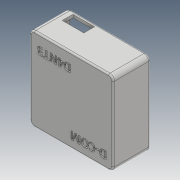
# Autodesk Inventor part: base
Saved by Autodesk Inventor 2017 (Build 210142000, 142)
## iProperties
Created: 2020-06-11
Part Number: base
Material: Generic
Document SubType Name: Modeling
Designer: c
Density: 1 g/cm^3
Appearance: Default
Author: c
Autodesk Inventor part; units mm, degrees
ref_plane "YZ Plane" through (0, 0, 0) normal (1, 0, 0) x (0, 1, 0)
ref_plane "XZ Plane" through (0, 0, 0) normal (0, 1, 0) x (-1, 0, 0)
ref_plane "XY Plane" through (0, 0, 0) normal (0, 0, 1) x (1, 0, 0)
sketch "Sketch1" plane through (0, 0, 0) normal (0, 1, 0) x (-1, 0, 0)
  line L0 (13, 15) -> (-37, 15)
  line L1 (-37, 15) -> (-37, -35)
  line L2 (-37, -35) -> (13, -35)
  line L3 (13, -35) -> (13, 15)
  line L4 (12, 17) -> (-36, 17)
  line L5 (-39, 14) -> (-39, -34)
  line L6 (-36, -37) -> (12, -37)
  line L7 (15, -34) -> (15, 14)
  arc A0 (15, 14) -> (12, 17) centre (12, 14) ccw
  arc A1 (-36, 17) -> (-39, 14) centre (-36, 14) ccw
  arc A2 (-39, -34) -> (-36, -37) centre (-36, -34) ccw
  arc A3 (12, -37) -> (15, -34) centre (12, -34) ccw
  point P0 (0, 0)
  dimension "d0" = 50
  dimension "d1" = 50
  dimension "d2" = 3
  constraints: 16 end point, 8 point on circle, 8 tangent, 4 centre point, 4 parallel, 3 equal radius, 2 perpendicular, 1 horizontal, 3 other
  measures "d0" distance of L2.end L1.end
  measures "d1" distance of L1.end L0.end
  measures "d2" radius of A0
extrude "Extrusion1" add sketch "Sketch1" along normal blind 24
sketch "Sketch2" plane through (0, 0, 0) normal (0, -1, 0) x (1, 0, 0)
  line L0 (36, 17) -> (-12, 17)
  line L1 (-15, 14) -> (-15, -34)
  line L2 (-12, -37) -> (36, -37)
  line L3 (39, -34) -> (39, 14)
  arc A0 (39, 14) -> (36, 17) centre (36, 14) ccw
  arc A1 (-12, 17) -> (-15, 14) centre (-12, 14) ccw
  arc A2 (-15, -34) -> (-12, -37) centre (-12, -34) ccw
  arc A3 (36, -37) -> (39, -34) centre (36, -34) ccw
  point P0 (0, 0)
  dimension "d5" = 3
  constraints: 8 end point, 8 point on circle, 8 tangent, 4 centre point, 3 equal radius, 2 parallel, 1 horizontal, 1 perpendicular
  measures "d5" radius of A0
extrude "Extrusion2" add sketch "Sketch2" against normal blind 2
fillet "Fillet1" radius 1 8 edges at (-14.1213, 0, 16.1213) (-15, 0, -10) (-14.1213, 0, -36.1213) (12, 0, -37) (38.1213, 0, -36.1213) (39, 0, -10) (38.1213, 0, 16.1213) (12, 0, 17)
sketch "Sketch3" plane through (36, 24, -37) normal (0, 0, -1) x (-1, 0, 0)
  line L0 (29, -12) -> (19, -12)
  line L1 (19, -12) -> (19, -8)
  line L2 (19, -8) -> (29, -8)
  line L3 (29, -8) -> (29, -12)
  line L4 (29, -18) -> (19, -18)
  line L5 (19, -18) -> (19, -14)
  line L6 (19, -14) -> (29, -14)
  line L7 (29, -14) -> (29, -18)
  line L8 (0, 0) -> (48, 0) projected
  line L9 (51, -23) -> (51, 0) projected
  line L10 (0, -24) -> (48, -24) projected
  point P0 (36, -24)
  dimension "d9" = 10
  dimension "d10" = 4
  dimension "d11" = 10
  dimension "d12" = 2
  dimension "d16" = 22
  dimension "d17" = 4
  dimension "d25" = 10
  constraints: 16 end point, 4 parallel, 2 horizontal, 2 perpendicular, 1 point on line
  measures "d9" distance of L1.end L2.end
  measures "d10" distance of L0.end L1.end
  measures "d11" distance of L5.end L6.end
  measures "d12" distance between parallel lines of L0 L6
  measures "d16" distance between parallel lines of L9 L7
  measures "d17" distance of L4.end L5.end
  measures "d25" distance between parallel lines of L10 L6
extrude "Extrusion3" cut sketch "Sketch3" against normal blind 4
sketch "Sketch4" plane through (0, 0, 0) normal (0, -1, 0) x (1, 0, 0)
  line L0 (11.8173, 5.1202) -> (-9.0886, 5.1202) construction
  line L1 (-9.0886, 5.1202) -> (-9.0886, 15.4837) construction
  line L2 (-9.0886, 15.4837) -> (11.8173, 15.4837) construction
  line L3 (11.8173, 15.4837) -> (11.8173, 5.1202) construction
  line L4 (34.9838, -32.0104) -> (14.0779, -32.0104) construction
  line L5 (14.0779, -32.0104) -> (14.0779, 11.03) construction
  line L6 (14.0779, 11.03) -> (34.9838, 11.03) construction
  line L7 (34.9838, 11.03) -> (34.9838, -32.0104) construction
  spline S0 degree 2 poles (7.1365, 7.6225) (7.1365, 8.3079) (7.4933, 9.2798) (8.1647, 9.8995) (9.1224, 10.1859) (9.7844, 10.1859) knots 0 0 0 1 2 3 4 4 4
  line L8 (9.7844, 10.1859) -> (10.9722, 10.1859)
  spline S1 degree 2 poles (10.9722, 10.1859) (11.0989, 10.1859) (11.2727, 10.0356) (11.2727, 9.8666) knots 0 0 0 1 2 2 2
  line L9 (11.2727, 9.8666) -> (11.2727, 5.5286)
  spline S2 degree 2 poles (11.2727, 5.5286) (11.2727, 5.3596) (11.0989, 5.2094) (10.9722, 5.2094) knots 0 0 0 1 2 2 2
  line L10 (10.9722, 5.2094) -> (9.6952, 5.2094)
  spline S3 degree 2 poles (9.6952, 5.2094) (9.0285, 5.2094) (8.1036, 5.5192) (7.4651, 6.1342) (7.1365, 7.031) (7.1365, 7.6225) knots 0 0 0 1 2 3 4 4 4
  spline S4 degree 2 poles (8.1835, 7.6601) (8.1835, 7.3079) (8.3478, 6.6976) (8.714, 6.2516) (9.2867, 6.0028) (9.7515, 6.0028) knots 0 0 0 1 2 3 4 4 4
  line L11 (9.7515, 6.0028) -> (10.2633, 6.0028)
  line L12 (10.2633, 6.0028) -> (10.2633, 9.3878)
  line L13 (10.2633, 9.3878) -> (9.7374, 9.3878)
  spline S5 degree 2 poles (9.7374, 9.3878) (9.3196, 9.3878) (8.7515, 9.1718) (8.3712, 8.7399) (8.1835, 8.092) (8.1835, 7.6601) knots 0 0 0 1 2 3 4 4 4
  spline S6 degree 2 poles (3.0144, 8.7587) (3.0144, 8.9558) (3.0942, 9.1577) (3.1647, 9.1577) knots 0 0 0 1 2 2 2
  line L14 (3.1647, 9.1577) -> (3.606, 9.1577)
  line L15 (3.606, 9.1577) -> (3.606, 10.0544)
  spline S7 degree 2 poles (3.606, 10.0544) (3.606, 10.092) (3.6529, 10.153) (3.7656, 10.1906) (3.9534, 10.2094) (4.0989, 10.2094) knots 0 0 0 1 2 3 4 4 4
  spline S8 degree 2 poles (4.0989, 10.2094) (4.2351, 10.2094) (4.4229, 10.1906) (4.5356, 10.153) (4.5778, 10.092) (4.5778, 10.0544) knots 0 0 0 1 2 3 4 4 4
  line L16 (4.5778, 10.0544) -> (4.5778, 9.1577)
  line L17 (4.5778, 9.1577) -> (6.4839, 9.1577)
  spline S9 degree 2 poles (6.4839, 9.1577) (6.5403, 9.1577) (6.6248, 9.1295) (6.6811, 9.0356) (6.7093, 8.8525) (6.7093, 8.7023) knots 0 0 0 1 2 3 4 4 4
  spline S10 degree 2 poles (6.7093, 8.7023) (6.7093, 8.5802) (6.6999, 8.4018) (6.6717, 8.2516) (6.6201, 8.1248) (6.5825, 8.0497) knots 0 0 0 1 2 3 4 4 4
  line L18 (6.5825, 8.0497) -> (5.0332, 5.322)
  spline S11 degree 2 poles (5.0332, 5.322) (5.0144, 5.2845) (4.9205, 5.2375) (4.7562, 5.2) (4.5027, 5.1859) (4.3196, 5.1859) knots 0 0 0 1 2 3 4 4 4
  spline S12 degree 2 poles (4.3196, 5.1859) (4.1224, 5.1859) (3.8501, 5.2047) (3.6811, 5.2469) (3.606, 5.3079) (3.606, 5.3502) knots 0 0 0 1 2 3 4 4 4
  line L19 (3.606, 5.3502) -> (3.606, 8.3502)
  line L20 (3.606, 8.3502) -> (3.1647, 8.3502)
  spline S13 degree 2 poles (3.1647, 8.3502) (3.1036, 8.3502) (3.0144, 8.538) (3.0144, 8.7587) knots 0 0 0 1 2 2 2
  line L21 (4.5778, 6.0591) -> (4.5872, 6.0591)
  line L22 (4.5872, 6.0591) -> (5.9018, 8.3502)
  line L23 (5.9018, 8.3502) -> (4.5778, 8.3502)
  line L24 (4.5778, 8.3502) -> (4.5778, 6.0591)
  spline S14 degree 2 poles (-1.7884, 9.8338) (-1.7884, 9.923) (-1.7273, 10.0591) (-1.6241, 10.153) (-1.4785, 10.1953) (-1.4081, 10.1953) knots 0 0 0 1 2 3 4 4 4
  line L25 (-1.4081, 10.1953) -> (-0.9762, 10.1953)
  spline S15 degree 2 poles (-0.9762, 10.1953) (-0.8447, 10.1953) (-0.6475, 10.1389) (-0.4832, 9.9981) (-0.3283, 9.754) (-0.2297, 9.5662) knots 0 0 0 1 2 3 4 4 4
  line L26 (-0.2297, 9.5662) -> (1.0097, 7.2375)
  spline S16 degree 2 poles (1.0097, 7.2375) (1.1177, 7.031) (1.3384, 6.5474) (1.4276, 6.322) knots 0 0 0 1 2 2 2
  line L27 (1.4276, 6.322) -> (1.437, 6.322)
  spline S17 degree 2 poles (1.437, 6.322) (1.4182, 6.599) (1.4041, 7.1483) (1.4041, 7.4394) knots 0 0 0 1 2 2 2
  line L28 (1.4041, 7.4394) -> (1.4041, 10.045)
  spline S18 degree 2 poles (1.4041, 10.045) (1.4041, 10.0826) (1.4464, 10.1436) (1.5496, 10.1859) (1.7281, 10.2094) (1.8642, 10.2094) knots 0 0 0 1 2 3 4 4 4
  spline S19 degree 2 poles (1.8642, 10.2094) (2.0004, 10.2094) (2.1788, 10.1859) (2.2773, 10.1436) (2.3149, 10.0826) (2.3149, 10.045) knots 0 0 0 1 2 3 4 4 4
  line L29 (2.3149, 10.045) -> (2.3149, 5.5709)
  spline S20 degree 2 poles (2.3149, 5.5709) (2.3149, 5.3878) (2.1036, 5.2094) (1.9487, 5.2094) knots 0 0 0 1 2 2 2
  line L30 (1.9487, 5.2094) -> (1.4088, 5.2094)
  spline S21 degree 2 poles (1.4088, 5.2094) (1.2633, 5.2094) (1.0614, 5.261) (0.9065, 5.3737) (0.7656, 5.5802) (0.6905, 5.7305) knots 0 0 0 1 2 3 4 4 4
  line L31 (0.6905, 5.7305) -> (-0.2766, 7.5474)
  spline S22 degree 2 poles (-0.2766, 7.5474) (-0.3611, 7.7164) (-0.5255, 8.0356) (-0.6804, 8.3549) (-0.8259, 8.6601) (-0.8964, 8.815) knots 0 0 0 1 2 3 4 4 4
  line L32 (-0.8964, 8.815) -> (-0.9011, 8.815)
  spline S23 degree 2 poles (-0.9011, 8.815) (-0.887, 8.5474) (-0.8776, 7.9605) (-0.8776, 7.6929) knots 0 0 0 1 2 2 2
  line L33 (-0.8776, 7.6929) -> (-0.8776, 5.3549)
  spline S24 degree 2 poles (-0.8776, 5.3549) (-0.8776, 5.3173) (-0.9245, 5.2563) (-1.0325, 5.2094) (-1.2062, 5.1906) (-1.3471, 5.1906) knots 0 0 0 1 2 3 4 4 4
  spline S25 degree 2 poles (-1.3471, 5.1906) (-1.4785, 5.1906) (-1.6522, 5.2094) (-1.7508, 5.2563) (-1.7884, 5.3173) (-1.7884, 5.3549) knots 0 0 0 1 2 3 4 4 4
  line L34 (-1.7884, 5.3549) -> (-1.7884, 9.8338)
  spline S26 degree 2 poles (-6.1781, 5.6225) (-6.1781, 5.7352) (-6.1593, 5.8948) (-6.1217, 5.9887) (-6.0607, 6.0356) (-6.0278, 6.0356) knots 0 0 0 1 2 3 4 4 4
  line L35 (-6.0278, 6.0356) -> (-4.7837, 6.0356)
  line L36 (-4.7837, 6.0356) -> (-4.7837, 10.0497)
  spline S27 degree 2 poles (-4.7837, 10.0497) (-4.7837, 10.0873) (-4.732, 10.1483) (-4.6194, 10.1859) (-4.4222, 10.2094) (-4.2766, 10.2094) knots 0 0 0 1 2 3 4 4 4
  spline S28 degree 2 poles (-4.2766, 10.2094) (-4.1311, 10.2094) (-3.9339, 10.1859) (-3.8212, 10.1483) (-3.7696, 10.0873) (-3.7696, 10.0497) knots 0 0 0 1 2 3 4 4 4
  line L37 (-3.7696, 10.0497) -> (-3.7696, 6.0356)
  line L38 (-3.7696, 6.0356) -> (-2.5255, 6.0356)
  spline S29 degree 2 poles (-2.5255, 6.0356) (-2.4879, 6.0356) (-2.4316, 5.9887) (-2.394, 5.8948) (-2.3752, 5.7352) (-2.3752, 5.6225) knots 0 0 0 1 2 3 4 4 4
  spline S30 degree 2 poles (-2.3752, 5.6225) (-2.3752, 5.5098) (-2.394, 5.3455) (-2.4316, 5.2516) (-2.4879, 5.2094) (-2.5255, 5.2094) knots 0 0 0 1 2 3 4 4 4
  line L39 (-2.5255, 5.2094) -> (-6.0278, 5.2094)
  spline S31 degree 2 poles (-6.0278, 5.2094) (-6.0607, 5.2094) (-6.1217, 5.2516) (-6.1593, 5.3455) (-6.1781, 5.5098) (-6.1781, 5.6225) knots 0 0 0 1 2 3 4 4 4
  spline S32 degree 2 poles (-9.887, 8.7305) (-9.887, 9.1014) (-9.6006, 9.6788) (-9.0935, 10.0732) (-8.3846, 10.2751) (-7.9668, 10.2751) knots 0 0 0 1 2 3 4 4 4
  spline S33 degree 2 poles (-7.9668, 10.2751) (-7.7133, 10.2751) (-7.2673, 10.2) (-6.9245, 10.0967) (-6.6992, 9.9793) (-6.6335, 9.9183) (-6.5959, 9.8385) (-6.5677, 9.7352) (-6.5583, 9.5802) (-6.5583, 9.4676) knots 0 0 0 1 2 3 4 5 6 7 8 8 8
  spline S34 degree 2 poles (-6.5583, 9.4676) (-6.5583, 9.2798) (-6.6194, 9.1389) (-6.6804, 9.1389) knots 0 0 0 1 2 2 2
  spline S35 degree 2 poles (-6.6804, 9.1389) (-6.718, 9.1389) (-6.9104, 9.2422) (-7.2015, 9.3643) (-7.5959, 9.4676) (-7.8447, 9.4676) knots 0 0 0 1 2 3 4 4 4
  spline S36 degree 2 poles (-7.8447, 9.4676) (-8.056, 9.4676) (-8.3799, 9.369) (-8.6053, 9.1859) (-8.718, 8.9277) (-8.718, 8.7727) knots 0 0 0 1 2 3 4 4 4
  spline S37 degree 2 poles (-8.718, 8.7727) (-8.718, 8.599) (-8.5818, 8.322) (-8.3189, 8.1248) (-7.9151, 8.0169) (-7.6381, 8.0169) knots 0 0 0 1 2 3 4 4 4
  line L40 (-7.6381, 8.0169) -> (-7.2062, 8.0169)
  spline S38 degree 2 poles (-7.2062, 8.0169) (-7.1593, 8.0169) (-7.0888, 7.9887) (-7.0419, 7.9042) (-7.0231, 7.754) (-7.0231, 7.6366) knots 0 0 0 1 2 3 4 4 4
  spline S39 degree 2 poles (-7.0231, 7.6366) (-7.0231, 7.5239) (-7.0419, 7.3831) (-7.0842, 7.3079) (-7.1499, 7.2751) (-7.1968, 7.2751) knots 0 0 0 1 2 3 4 4 4
  line L41 (-7.1968, 7.2751) -> (-7.6335, 7.2751)
  spline S40 degree 2 poles (-7.6335, 7.2751) (-7.8588, 7.2751) (-8.2062, 7.1718) (-8.441, 6.9793) (-8.563, 6.707) (-8.563, 6.538) knots 0 0 0 1 2 3 4 4 4
  spline S41 degree 2 poles (-8.563, 6.538) (-8.563, 6.4112) (-8.4785, 6.1859) (-8.3142, 6.0216) (-8.0513, 5.923) (-7.8729, 5.923) knots 0 0 0 1 2 3 4 4 4
  spline S42 degree 2 poles (-7.8729, 5.923) (-7.671, 5.923) (-7.3189, 6.0403) (-7.0372, 6.1859) (-6.84, 6.3079) (-6.7931, 6.3079) knots 0 0 0 1 2 3 4 4 4
  spline S43 degree 2 poles (-6.7931, 6.3079) (-6.7649, 6.3079) (-6.718, 6.2798) (-6.6851, 6.2047) (-6.671, 6.0591) (-6.671, 5.9417) knots 0 0 0 1 2 3 4 4 4
  spline S44 degree 2 poles (-6.671, 5.9417) (-6.671, 5.8479) (-6.6804, 5.7211) (-6.7039, 5.6366) (-6.7367, 5.5756) (-6.8119, 5.5004) (-7.0513, 5.3549) (-7.4128, 5.214) (-7.887, 5.1202) (-8.164, 5.1202) knots 0 0 0 1 2 3 4 5 6 7 8 8 8
  spline S45 degree 2 poles (-8.164, 5.1202) (-8.5255, 5.1202) (-9.0842, 5.2892) (-9.4644, 5.6084) (-9.6616, 6.0732) (-9.6616, 6.369) knots 0 0 0 1 2 3 4 4 4
  spline S46 degree 2 poles (-9.6616, 6.369) (-9.6616, 6.5943) (-9.5442, 6.984) (-9.3236, 7.2939) (-8.9856, 7.5098) (-8.7696, 7.5615) knots 0 0 0 1 2 3 4 4 4
  line L42 (-8.7696, 7.5615) -> (-8.7696, 7.5756)
  spline S47 degree 2 poles (-8.7696, 7.5756) (-9.0278, 7.6037) (-9.4457, 7.8103) (-9.732, 8.1155) (-9.887, 8.5051) (-9.887, 8.7305) knots 0 0 0 1 2 3 4 4 4
  spline S48 degree 2 poles (30.303, -29.5081) (30.303, -28.8226) (30.6598, -27.8508) (31.3312, -27.2311) (32.2889, -26.9447) (32.9509, -26.9447) knots 0 0 0 1 2 3 4 4 4
  line L43 (32.9509, -26.9447) -> (34.1387, -26.9447)
  spline S49 degree 2 poles (34.1387, -26.9447) (34.2654, -26.9447) (34.4392, -27.0949) (34.4392, -27.2639) knots 0 0 0 1 2 2 2
  line L44 (34.4392, -27.2639) -> (34.4392, -31.602)
  spline S50 degree 2 poles (34.4392, -31.602) (34.4392, -31.771) (34.2654, -31.9212) (34.1387, -31.9212) knots 0 0 0 1 2 2 2
  line L45 (34.1387, -31.9212) -> (32.8617, -31.9212)
  spline S51 degree 2 poles (32.8617, -31.9212) (32.195, -31.9212) (31.2701, -31.6114) (30.6316, -30.9963) (30.303, -30.0996) (30.303, -29.5081) knots 0 0 0 1 2 3 4 4 4
  spline S52 degree 2 poles (31.35, -29.4705) (31.35, -29.8226) (31.5143, -30.433) (31.8805, -30.879) (32.4532, -31.1278) (32.918, -31.1278) knots 0 0 0 1 2 3 4 4 4
  line L46 (32.918, -31.1278) -> (33.4298, -31.1278)
  line L47 (33.4298, -31.1278) -> (33.4298, -27.7428)
  line L48 (33.4298, -27.7428) -> (32.9039, -27.7428)
  spline S53 degree 2 poles (32.9039, -27.7428) (32.4861, -27.7428) (31.918, -27.9588) (31.5377, -28.3907) (31.35, -29.0386) (31.35, -29.4705) knots 0 0 0 1 2 3 4 4 4
  spline S54 degree 2 poles (27.8335, -28.879) (27.8335, -28.6583) (27.918, -28.4799) (28.0119, -28.4799) knots 0 0 0 1 2 2 2
  line L49 (28.0119, -28.4799) -> (29.6082, -28.4799)
  spline S55 degree 2 poles (29.6082, -28.4799) (29.7068, -28.4799) (29.7913, -28.663) (29.7913, -28.879) knots 0 0 0 1 2 2 2
  spline S56 degree 2 poles (29.7913, -28.879) (29.7913, -29.0949) (29.7068, -29.2733) (29.6082, -29.2733) knots 0 0 0 1 2 2 2
  line L50 (29.6082, -29.2733) -> (28.0119, -29.2733)
  spline S57 degree 2 poles (28.0119, -29.2733) (27.965, -29.2733) (27.8992, -29.2358) (27.8523, -29.1419) (27.8335, -28.9869) (27.8335, -28.879) knots 0 0 0 1 2 3 4 4 4
  spline S58 degree 2 poles (23.6176, -27.7006) (23.6176, -27.6067) (23.6269, -27.4705) (23.6504, -27.3766) (23.6927, -27.3062) (23.7772, -27.217) (24.0166, -27.0761) (24.3687, -26.9494) (24.8194, -26.8649) (25.0777, -26.8649) knots 0 0 0 1 2 3 4 5 6 7 8 8 8
  spline S59 degree 2 poles (25.0777, -26.8649) (25.5894, -26.8649) (26.4157, -27.1794) (26.9885, -27.8085) (27.2983, -28.7428) (27.2983, -29.3672) knots 0 0 0 1 2 3 4 4 4
  spline S60 degree 2 poles (27.2983, -29.3672) (27.2983, -30.001) (26.9603, -30.9869) (26.35, -31.6536) (25.5002, -32.001) (24.9885, -32.001) knots 0 0 0 1 2 3 4 4 4
  spline S61 degree 2 poles (24.9885, -32.001) (24.7819, -32.001) (24.3969, -31.9306) (24.0683, -31.8179) (23.81, -31.6724) (23.7068, -31.5691) (23.6645, -31.4987) (23.641, -31.3907) (23.6316, -31.2452) (23.6316, -31.1372) knots 0 0 0 1 2 3 4 5 6 7 8 8 8
  spline S62 degree 2 poles (23.6316, -31.1372) (23.6316, -31.0245) (23.6457, -30.8602) (23.6833, -30.7616) (23.7396, -30.7146) (23.7725, -30.7146) knots 0 0 0 1 2 3 4 4 4
  spline S63 degree 2 poles (23.7725, -30.7146) (23.8335, -30.7146) (24.0072, -30.8508) (24.2889, -31.0151) (24.6786, -31.1513) (24.9462, -31.1513) knots 0 0 0 1 2 3 4 4 4
  spline S64 degree 2 poles (24.9462, -31.1513) (25.242, -31.1513) (25.7068, -30.9071) (26.0354, -30.4611) (26.2044, -29.8226) (26.2044, -29.4236) knots 0 0 0 1 2 3 4 4 4
  spline S65 degree 2 poles (26.2044, -29.4236) (26.2044, -28.9822) (26.026, -28.3437) (25.688, -27.9259) (25.2185, -27.724) (24.9227, -27.724) knots 0 0 0 1 2 3 4 4 4
  spline S66 degree 2 poles (24.9227, -27.724) (24.6504, -27.724) (24.2608, -27.8508) (23.9791, -28.0057) (23.796, -28.1278) (23.749, -28.1278) knots 0 0 0 1 2 3 4 4 4
  spline S67 degree 2 poles (23.749, -28.1278) (23.7115, -28.1278) (23.6645, -28.0949) (23.6316, -28.0057) (23.6176, -27.8414) (23.6176, -27.7006) knots 0 0 0 1 2 3 4 4 4
  spline S68 degree 2 poles (18.411, -29.4893) (18.411, -28.8696) (18.7208, -27.893) (19.3265, -27.2123) (20.2232, -26.8555) (20.81, -26.8555) knots 0 0 0 1 2 3 4 4 4
  spline S69 degree 2 poles (20.81, -26.8555) (21.3922, -26.8555) (22.2608, -27.1607) (22.8382, -27.7804) (23.1246, -28.7428) (23.1246, -29.4001) knots 0 0 0 1 2 3 4 4 4
  spline S70 degree 2 poles (23.1246, -29.4001) (23.1246, -30.0057) (22.8147, -30.9729) (22.2091, -31.6489) (21.3124, -32.0104) (20.7208, -32.0104) knots 0 0 0 1 2 3 4 4 4
  spline S71 degree 2 poles (20.7208, -32.0104) (20.1528, -32.0104) (19.2889, -31.7099) (18.7068, -31.0855) (18.411, -30.1372) (18.411, -29.4893) knots 0 0 0 1 2 3 4 4 4
  spline S72 degree 2 poles (19.472, -29.4376) (19.472, -29.8273) (19.5941, -30.4705) (19.8899, -30.9306) (20.3828, -31.1794) (20.7537, -31.1794) knots 0 0 0 1 2 3 4 4 4
  spline S73 degree 2 poles (20.7537, -31.1794) (21.1293, -31.1794) (21.6269, -30.8977) (21.9368, -30.4283) (22.0636, -29.8038) (22.0636, -29.4517) knots 0 0 0 1 2 3 4 4 4
  spline S74 degree 2 poles (22.0636, -29.4517) (22.0636, -29.0433) (21.9415, -28.3954) (21.6457, -27.9353) (21.1528, -27.6912) (20.7819, -27.6912) knots 0 0 0 1 2 3 4 4 4
  spline S75 degree 2 poles (20.7819, -27.6912) (20.4063, -27.6912) (19.9086, -27.9682) (19.5988, -28.447) (19.472, -29.0808) (19.472, -29.4376) knots 0 0 0 1 2 3 4 4 4
  spline S76 degree 2 poles (11.7584, -27.0808) (11.7584, -27.0433) (11.8007, -26.9822) (11.9133, -26.9447) (12.0964, -26.9212) (12.2373, -26.9212) knots 0 0 0 1 2 3 4 4 4
  spline S77 degree 2 poles (12.2373, -26.9212) (12.3781, -26.9212) (12.5612, -26.9447) (12.6692, -26.9822) (12.7162, -27.0433) (12.7162, -27.0808) knots 0 0 0 1 2 3 4 4 4
  line L51 (12.7162, -27.0808) -> (12.7162, -31.1325)
  line L52 (12.7162, -31.1325) -> (12.7255, -31.1325)
  line L53 (12.7255, -31.1325) -> (14.1669, -27.0855)
  spline S78 degree 2 poles (14.1669, -27.0855) (14.1809, -27.0386) (14.2514, -26.9729) (14.3687, -26.9306) (14.5565, -26.9212) (14.688, -26.9212) knots 0 0 0 1 2 3 4 4 4
  spline S79 degree 2 poles (14.688, -26.9212) (14.8147, -26.9212) (15.0025, -26.94) (15.1199, -26.9822) (15.1903, -27.0433) (15.1997, -27.0855) knots 0 0 0 1 2 3 4 4 4
  line L54 (15.1997, -27.0855) -> (16.5941, -31.1325)
  line L55 (16.5941, -31.1325) -> (16.6035, -31.1325)
  line L56 (16.6035, -31.1325) -> (16.6035, -27.0808)
  spline S80 degree 2 poles (16.6035, -27.0808) (16.6035, -27.0433) (16.6457, -26.9822) (16.7631, -26.9447) (16.9415, -26.9212) (17.0823, -26.9212) knots 0 0 0 1 2 3 4 4 4
  spline S81 degree 2 poles (17.0823, -26.9212) (17.2232, -26.9212) (17.4063, -26.9447) (17.519, -26.9822) (17.5612, -27.0433) (17.5612, -27.0808) knots 0 0 0 1 2 3 4 4 4
  line L57 (17.5612, -27.0808) -> (17.5612, -31.5175)
  spline S82 degree 2 poles (17.5612, -31.5175) (17.5612, -31.7146) (17.3546, -31.9212) (17.1809, -31.9212) knots 0 0 0 1 2 2 2
  line L58 (17.1809, -31.9212) -> (16.519, -31.9212)
  spline S83 degree 2 poles (16.519, -31.9212) (16.3406, -31.9212) (16.087, -31.8649) (15.9039, -31.7287) (15.7819, -31.5081) (15.7349, -31.3484) knots 0 0 0 1 2 3 4 4 4
  line L59 (15.7349, -31.3484) -> (14.6551, -28.3813)
  line L60 (14.6551, -28.3813) -> (14.641, -28.3813)
  line L61 (14.641, -28.3813) -> (13.5237, -31.3391)
  spline S84 degree 2 poles (13.5237, -31.3391) (13.472, -31.5034) (13.3546, -31.724) (13.195, -31.8649) (12.9838, -31.9212) (12.8382, -31.9212) knots 0 0 0 1 2 3 4 4 4
  line L62 (12.8382, -31.9212) -> (12.1575, -31.9212)
  spline S85 degree 2 poles (12.1575, -31.9212) (12.0542, -31.9212) (11.9039, -31.8696) (11.81, -31.7616) (11.7584, -31.6114) (11.7584, -31.5175) knots 0 0 0 1 2 3 4 4 4
  line L63 (11.7584, -31.5175) -> (11.7584, -27.0808)
  point P0 (0, 0)
  constraints: 4 other
emboss "Emboss1" sketch "Sketch4" operation cut depth 1 direction (0, 1, 0)
sketch "Sketch5" plane through (-12, 24, 17) normal (0, 0, 1) x (1, 0, 0)
  line L0 (29, -12) -> (29, -8) projected
  line L1 (17, -9) -> (2.9977, -9)
  line L2 (2.9977, -9) -> (2.9977, -2)
  line L3 (2.9977, -2) -> (17, -2)
  line L4 (17, -2) -> (17, -9)
  line L5 (-3, -23) -> (-3, 0) projected
  line L6 (0, -24) -> (48, -24) projected
  point P0 (12, -24)
  dimension "d26" = 20
  dimension "d27" = 15
  dimension "d28" = 7
  constraints: 8 end point, 2 parallel, 1 horizontal, 1 perpendicular
  measures "d26" distance between parallel lines of L5 L4
  measures "d27" distance between parallel lines of L6 L1
  measures "d28" distance between parallel lines of L1 L3
extrude "Extrusion4" cut sketch "Sketch5" against normal blind 4
fillet "Fillet2" radius 1 8 edges at (38.1213, 24, 16.1213) (39, 24, -10) (38.1213, 24, -36.1213) (12, 24, -37) (-14.1213, 24, -36.1213) (-15, 24, -10) (-14.1213, 24, 16.1213) (12, 24, 17)
sketch "Sketch6" plane through (36, 1, -37) normal (0, 0, -1) x (-1, 0, 0)
  line L0 (11.499, 15.0896) -> (15.0018, 15.0896) construction
  line L1 (15.0018, 15.0896) -> (15.0018, 12.3412) construction
  line L2 (15.0018, 12.3412) -> (11.499, 12.3412) construction
  line L3 (11.499, 12.3412) -> (11.499, 15.0896) construction
  line L4 (12.8015, 7.2924) -> (14.6948, 7.2924) construction
  line L5 (14.6948, 7.2924) -> (14.6948, 1.0271) construction
  line L6 (14.6948, 1.0271) -> (12.8015, 1.0271) construction
  line L7 (12.8015, 1.0271) -> (12.8015, 7.2924) construction
  line L8 (15.9763, 12.857) -> (14.2826, 12.857)
  line L9 (14.2826, 12.857) -> (14.2826, 11.1633)
  line L10 (14.2826, 11.1633) -> (13.7234, 11.1633)
  line L11 (13.7234, 11.1633) -> (13.7234, 12.857)
  line L12 (13.7234, 12.857) -> (12.0298, 12.857)
  line L13 (12.0298, 12.857) -> (12.0298, 13.3959)
  line L14 (12.0298, 13.3959) -> (13.7234, 13.3959)
  line L15 (13.7234, 13.3959) -> (13.7234, 15.0896)
  line L16 (13.7234, 15.0896) -> (14.2826, 15.0896)
  line L17 (14.2826, 15.0896) -> (14.2826, 13.3959)
  line L18 (14.2826, 13.3959) -> (15.9763, 13.3959)
  line L19 (15.9763, 13.3959) -> (15.9763, 12.857)
  line L20 (14.9976, 6.6846) -> (13.1054, 6.6846)
  line L21 (13.1054, 6.6846) -> (13.1054, 7.2924)
  line L22 (13.1054, 7.2924) -> (14.9976, 7.2924)
  line L23 (14.9976, 7.2924) -> (14.9976, 6.6846)
  point P0 (36, -1)
  constraints: 4 other
emboss "Emboss2" sketch "Sketch6" operation cut depth 1 direction (0, 0, 1)
body "Solid1"
